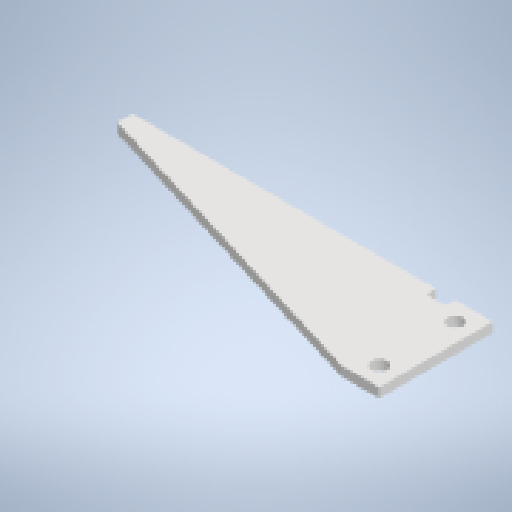
# Autodesk Inventor part: Gripper triangle
Saved by Autodesk Inventor 2023 (Build 270158000, 158)
## iProperties
Created: 2023-02-27
Part Number: Gripper triangle
Material: Generic
Document SubType Name: Modeling
Designer: Gabriel - T3 CAD
Density: 1 g/cm^3
Appearance: Default
Author: Gabriel - T3 CAD
Autodesk Inventor part; units mm, degrees
ref_plane "YZ Plane" through (0, 0, 0) normal (1, 0, 0) x (0, 1, 0)
ref_plane "XZ Plane" through (0, 0, 0) normal (0, 1, 0) x (-1, 0, 0)
ref_plane "XY Plane" through (0, 0, 0) normal (0, 0, 1) x (1, 0, 0)
sketch "Sketch1" plane through (0, 0, 0) normal (0, 1, 0) x (-1, 0, 0)
  line L0 (0, 0) -> (12.7, 0)
  line L1 (12.7, 0) -> (12.7, 38.1)
  line L2 (12.7, 38.1) -> (0, 38.1)
  line L3 (0, 38.1) -> (0, 0)
  circle A0 centre (6.35, 31.75) radius 2.5797
  circle A1 centre (6.35, 6.35) radius 2.5797
  line L4 (0, 0) -> (127, 0)
  line L5 (127, 0) -> (127, 3.175)
  line L6 (127, 3.175) -> (0, 3.175)
  line L7 (0, 3.175) -> (0, 0)
  line L8 (12.7, 38.1) -> (127, 3.175)
  line L9 (0, 3.175) -> (127, 3.175)
  line L10 (127, 3.175) -> (127, 1.5875)
  line L11 (127, 1.5875) -> (0, 1.5875)
  line L12 (0, 1.5875) -> (0, 3.175)
  line L13 (0, 3.175) -> (19.05, 3.175)
  line L14 (19.05, 3.175) -> (19.05, 1.5875)
  line L15 (19.05, 1.5875) -> (0, 1.5875)
  line L16 (0, 1.5875) -> (0, 3.175)
  line L17 (127, 3.175) -> (120.65, 3.175)
  line L18 (120.65, 3.175) -> (120.65, 1.5875)
  line L19 (120.65, 1.5875) -> (127, 1.5875)
  line L20 (127, 1.5875) -> (127, 3.175)
  line L21 (120.65, 3.175) -> (120.65, 5.1153)
  line L22 (127, 0) -> (0, 0)
  line L23 (0, 0) -> (0, -12.7)
  line L24 (0, -12.7) -> (127, -12.7)
  line L25 (127, -12.7) -> (127, 0)
  line L26 (120.65, 1.5875) -> (120.65, 0)
  line L27 (19.05, 1.5875) -> (19.05, 0)
  point P0 (0, 3.175)
  point P1 (0, 1.5875)
  point P2 (120.65, 1.5875)
  point P3 (120.65, 3.175)
  point P4 (19.05, 3.175)
  point P5 (19.05, 1.5875)
  point P6 (120.65, 3.175)
  point P7 (12.7, 1.5875)
  point P8 (12.7, 3.175)
  dimension "d0" = 12.7
  dimension "d1" = 6.35
  dimension "d2" = 6.35
  dimension "d3" = 25.4
  dimension "d5" = 6.35
  dimension "d6" = 5.1594
  dimension "d7" = 127
  dimension "d8" = 3.175
  dimension "d9" = 127
  dimension "d10" = 1.5875
  dimension "d15" = 19.05
  dimension "d16" = 1.5875
  dimension "d17" = 6.35
  dimension "d18" = 1.5875
  dimension "d25" = 12.7
  dimension "d27" = 6.35
  constraints: 56 end point, 12 parallel, 8 perpendicular, 5 horizontal, 3 point on line, 2 centre point, 1 equal radius, 1 vertical
  measures "d0" distance of L2.end L1.end
  measures "d1" distance from line of L3 A0.centre
  measures "d2" distance from line of L3 A1.centre
  measures "d3" distance of A1.centre A0.centre
  measures "d5" distance from line of L2 A0.centre
  measures "d6" diameter of A0
  measures "d7" distance of L6.end L5.end
  measures "d8" distance of L5.end L4.end
  measures "d9" distance of L10.end L11.end
  measures "d10" distance of L9.end L10.end
  measures "d15" distance of L14.end L15.end
  measures "d16" distance of L13.end L14.end
  measures "d17" distance of L19.end L18.end
  measures "d18" distance of L18.end L17.end
  measures "d25" distance between parallel lines of L4 L24
  measures "d27" distance from line of L4 A1.centre
extrude "Extrusion1" add sketch "Sketch1" along normal blind 3.175 contours L3 L11 L1 L0 | L3 L6 L1 L11 | L3 L2 L1 L6 | L1 L8 L21 L6
extrude "Extrusion2" add sketch "Sketch1" along normal up to surface (3.175 mm away) contours L27 L11 L26 L4 | L14 L6 L18 L11
fillet "Fillet1" radius 3.175 3 edges at (-12.7, 1.5875, 0) (0, 1.5875, 0) (0, 1.5875, 38.1)
equation "\"d1\" = d5"
equation "\"d2\" = d21"
equation "\"d5\" = 0.5 * d0"
equation "\"d16\" = d18"
equation "\"d21\" = d5"
body "Solid1"
